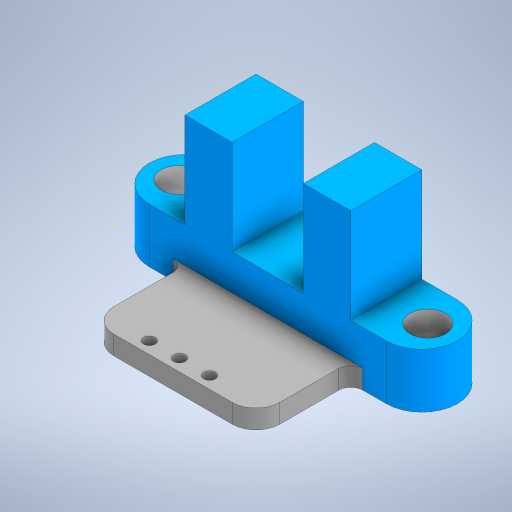
# Autodesk Inventor part: optocoupler
Saved by Autodesk Inventor 2023 (Build 270158000, 158)
## iProperties
Created: 2023-10-19
Part Number: optocoupler
Material: Generic
Document SubType Name: Modeling
Designer: mark
Density: 1 g/cm^3
Appearance: Default
Author: mark
Autodesk Inventor part; units mm, degrees
ref_plane "YZ Plane" through (0, 0, 0) normal (1, 0, 0) x (0, 1, 0)
ref_plane "XZ Plane" through (0, 0, 0) normal (0, 1, 0) x (-1, 0, 0)
ref_plane "XY Plane" through (0, 0, 0) normal (0, 0, 1) x (1, 0, 0)
sketch "Sketch1" plane through (0, 0, 0) normal (0, 1, 0) x (-1, 0, 0)
  line L0 (-3, 0) -> (-23, 0)
  line L1 (-26, -3) -> (-26, -3)
  line L2 (-23, -6) -> (-3, -6)
  line L3 (0, -3) -> (0, -3)
  arc A0 (-3, -6) -> (0, -3) centre (-3, -3) ccw
  arc A1 (0, -3) -> (-3, 0) centre (-3, -3) ccw
  arc A2 (-23, 0) -> (-26, -3) centre (-23, -3) ccw
  arc A3 (-26, -3) -> (-23, -6) centre (-23, -3) ccw
  circle A4 centre (-2.5, -3) radius 1.5
  circle A5 centre (-23.5, -3) radius 1.5
  point P0 (0, 0)
  point P1 (-26, -6)
  point P2 (-26, 0)
  point P3 (0, -6)
  dimension "d0" = 26
  dimension "d1" = 6
  dimension "d2" = 3
  dimension "d20" = 3
  dimension "d21" = 3
  dimension "d22" = 2.5
  dimension "d23" = 2.5
  constraints: 8 end point, 8 point on circle, 8 point on line, 8 tangent, 6 centre point, 3 equal radius, 2 parallel, 1 horizontal, 1 perpendicular
  measures "d0" distance of point (0, -6) point (-26, -6)
  measures "d1" distance of point (-26, -6) point (-26, 0)
  measures "d2" radius of A0
  measures "d20" diameter of A4
  measures "d21" diameter of A5
  measures "d22" horizontal distance of point (0, 0) A4.centre
  measures "d23" horizontal distance of A5.centre point (-26, 0)
extrude "Extrusion1" add sketch "Sketch1" along normal blind 3
sketch "Sketch2" plane through (0, 3, 0) normal (0, 1, 0) x (1, 0, 0)
  line L0 (3, 0) -> (23, 0) projected
  line L1 (23, 6) -> (3, 6) projected
  line L2 (6, 0) -> (10, 0)
  line L3 (10, 0) -> (10, 6)
  line L4 (10, 6) -> (6, 6)
  line L5 (6, 6) -> (6, 0)
  line L6 (16, 6) -> (20, 6)
  line L7 (20, 6) -> (20, 0)
  line L8 (20, 0) -> (16, 0)
  line L9 (16, 0) -> (16, 6)
  arc A0 (3, 6) -> (3, 0) centre (3, 3) ccw projected
  point P0 (0, 0)
  point P1 (0, 3)
  point P2 (20, 0)
  dimension "d5" = 4
  dimension "d6" = 4
  dimension "d7" = 6
  dimension "d8" = 6
  constraints: 16 end point, 4 parallel, 4 point on line, 2 horizontal, 2 perpendicular, 1 point on circle
  measures "d5" distance of L4.end L3.end
  measures "d6" distance of L7.end L8.end
  measures "d7" distance between parallel lines of L9 L3
  measures "d8" distance from line of point (0, 3) L5
extrude "Extrusion2" add sketch "Sketch2" along normal blind 8 contours L5 L1 L3 L0 | L9 L1 L7 L0
sketch "Sketch4" plane through (0, 0, 0) normal (0, -1, 0) x (1, 0, 0)
  point P0 (0, 0)
extrude "Extrusion4" add sketch "Sketch1" against normal blind 1.6
sketch "Sketch5" plane through (10, 3, 0) normal (0, 0, 1) x (1, 0, 0)
  line L0 (13, -4.6) -> (-7, -4.6) projected
  line L1 (-4, -4.6) -> (10, -4.6)
  line L2 (10, -4.6) -> (10, -3)
  line L3 (10, -3) -> (-4, -3)
  line L4 (-4, -3) -> (-4, -4.6)
  line L5 (10, 0) -> (10, 8) projected
  point P0 (-10, -3)
  point P1 (10, -4.6)
  dimension "d26" = 14
  dimension "d27" = 0
  constraints: 8 end point, 2 parallel, 1 horizontal, 1 perpendicular, 1 point on line
  measures "d26" distance of L3.end L2.end
  measures "d27" distance between parallel lines of L5 L2
extrude "Extrusion5" add sketch "Sketch5" along normal blind 8
fillet "Fillet1" radius 2 2 edges at (6, -0.8, 8) (20, -0.8, 8)
fillet "Fillet1" radius 1 2 edges at (6, -0.8, 0) (20, -0.8, 0)
sketch "Sketch6" plane through (5, 0, 0) normal (0, 1, 0) x (1, 0, 0)
  circle A0 centre (5, -7) radius 0.5
  circle A1 centre (7.54, -7) radius 0.5
  circle A2 centre (10.08, -7) radius 0.5
  line L0 (1, -1) -> (1, -6) projected
  line L1 (13, -8) -> (3, -8) projected
  point P0 (-5, 0)
  dimension "d32" = 1
  dimension "d33" = 1
  dimension "d34" = 1
  dimension "d36" = 2.54
  dimension "d37" = 2.54
  dimension "d38" = 4
  dimension "d39" = 0
  dimension "d40" = 1
  dimension "d41" = 1
  constraints: 3 centre point
  measures "d32" diameter of A0
  measures "d33" diameter of A1
  measures "d34" diameter of A2
  measures "d36" distance of A1.centre A0.centre
  measures "d37" distance of A2.centre A1.centre
  measures "d38" distance from line of L0 A0.centre
  measures "d39" vertical distance of A0.centre A1.centre
  measures "d40" distance from line of L1 A0.centre
  measures "d41" distance from line of L1 A2.centre
extrude "Extrusion6" cut sketch "Sketch6" against normal blind 8
equation "\"d37\" = d36"
equation "\"d41\" = d40"
body "Solid1"
